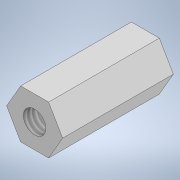
# Autodesk Inventor part: magneet stand-offs16 mm
Saved by Autodesk Inventor 2021 (Build 250183000, 183)
## iProperties
Created: 2023-11-13
Part Number: magneet stand-offs16 mm
Material: Generic
Document SubType Name: Modeling
Designer: Elias
Density: 1 g/cm^3
Appearance: Default
Author: Elias
Autodesk Inventor part; units mm, degrees
ref_plane "YZ Plane" through (0, 0, 0) normal (1, 0, 0) x (0, 1, 0)
ref_plane "XZ Plane" through (0, 0, 0) normal (0, 1, 0) x (-1, 0, 0)
ref_plane "XY Plane" through (0, 0, 0) normal (0, 0, 1) x (1, 0, 0)
sketch "Sketch1" plane through (0, 0, 0) normal (0, 0, 1) x (1, 0, 0)
  line L0 (4.0415, 0) -> (2.0207, -3.5)
  line L1 (2.0207, -3.5) -> (-2.0207, -3.5)
  line L2 (-2.0207, -3.5) -> (-4.0415, 0)
  line L3 (-4.0415, 0) -> (-2.0207, 3.5)
  line L4 (-2.0207, 3.5) -> (2.0207, 3.5)
  line L5 (2.0207, 3.5) -> (4.0415, 0)
  point P0 (0, 0)
  point P1 (0, 0)
  dimension "d0" = 7
  constraints: 12 end point, 1 coincident, 13 other
  measures "d0" distance between parallel lines of L2 L5
extrude "Extrusion1" add sketch "Sketch1" along normal blind 16
sketch "Sketch2" plane through (0, 0, 16) normal (0, 0, 1) x (1, 0, 0)
  point P0 (0, 0)
  point P1 (0, 0)
  constraints: 1 coincident
hole "Hole1" at (0, 0, 16) direction (0, 0, -1) diameter 3.242 depth 11.8 thread size "M4x0.7" class "6H" standard "ISO Metric profile"
body "Solid1"
